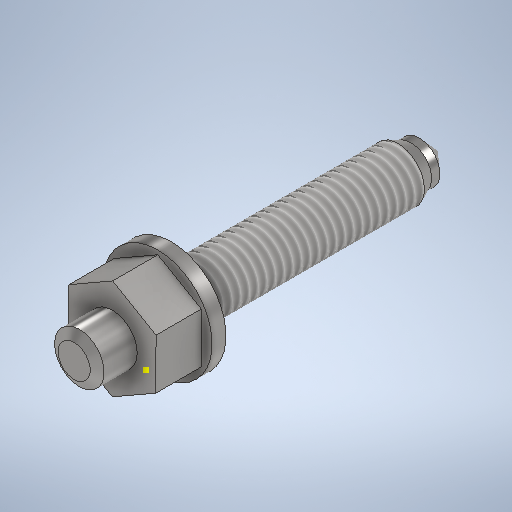
# Autodesk Inventor part: śróbki1
Saved by Autodesk Inventor 2025 (Build 290162000, 162)
## iProperties
Created: 2025-03-16
Part Number: śróbki1
Material: Stal nierdzewna
Document SubType Name: Modeling
Designer: barte
Density: 8 g/cm^3
Appearance: Częściowo polerowany
Author: barte
Autodesk Inventor part; units mm, degrees
ref_plane "YZ Plane" through (0, 0, 0) normal (1, 0, 0) x (0, 1, 0)
ref_plane "XZ Plane" through (0, 0, 0) normal (0, 1, 0) x (-1, 0, 0)
ref_plane "XY Plane" through (0, 0, 0) normal (0, 0, 1) x (1, 0, 0)
sketch "Szkic1" plane through (0, 0, 0) normal (0, 1, 0) x (-1, 0, 0)
  line L0 (0, 3.2611) -> (1.85, 3.2611)
  line L1 (1.85, 3.2611) -> (2.85, 2.6611)
  line L2 (2.85, 2.6611) -> (2.85, -6.3389)
  line L3 (2.85, -6.3389) -> (6.25, -6.3389)
  line L4 (6.25, -6.3389) -> (6.25, -7.9389)
  line L5 (6.25, -7.9389) -> (3.05, -7.9389)
  line L6 (3.05, -7.9389) -> (3.05, -33.9389)
  line L7 (3.05, -33.9389) -> (2.38, -35.4389)
  line L8 (2.38, -35.4389) -> (2.38, -36.3889)
  line L9 (2.38, -36.3889) -> (0, -38.5259)
  line L10 (0, 3.2611) -> (0, -38.5259)
  point P0 (0, 0)
  dimension "d0" = 1.85
  dimension "d1" = 0.6
  dimension "d2" = 1
  dimension "d3" = 9
  dimension "d4" = 3.4
  dimension "d5" = 1.6
  dimension "d6" = 3.2
  dimension "d7" = 26
  dimension "d8" = 1.5
  dimension "d9" = 0.67
  dimension "d10" = 0.95
  dimension "d11" = 2.137
  constraints: 22 end point, 3 perpendicular, 3 vertical, 2 horizontal
  measures "d0" distance of L0.start L0.end
  measures "d1" vertical distance of L0.end L1.end
  measures "d2" horizontal distance of L1.end L0.end
  measures "d3" distance of L1.end L2.end
  measures "d4" distance of L2.end L3.end
  measures "d5" distance of L3.end L4.end
  measures "d6" distance of L4.end L5.end
  measures "d7" distance of L5.end L6.end
  measures "d8" vertical distance of L6.end L7.end
  measures "d9" horizontal distance of L7.end L6.end
  measures "d10" distance of L7.end L8.end
  measures "d11" vertical distance of L9.end L8.end
revolve "Obrót1" add sketch "Szkic1" angle 360 about axis through (0, 0, 3.2611) along (0, 0, -1)
sketch "Szkic2" plane through (0, 0, -6.3389) normal (0, 0, 1) x (1, 0, 0)
  circle A0 centre (0, 0) radius 1.85 projected
  line L0 (5.0074, 2.8738) -> (4.9925, -2.8997)
  line L1 (4.9925, -2.8997) -> (-0.0149, -5.7735)
  line L2 (-0.0149, -5.7735) -> (-5.0074, -2.8738)
  line L3 (-5.0074, -2.8738) -> (-4.9925, 2.8997)
  line L4 (-4.9925, 2.8997) -> (0.0149, 5.7735)
  line L5 (0.0149, 5.7735) -> (5.0074, 2.8738)
  circle A1 centre (0, 0) radius 5
  point P0 (0, 0)
  dimension "d13" = 10
  constraints: 12 end point, 2 coincident, 1 centre point, 1 tangent, 13 other
  measures "d13" distance between parallel lines of L0 L3
sketch "Szkic3" plane through (0, 0, -7.9389) normal (0, 0, -1) x (-1, 0, 0)
  point P0 (0, 0)
extrude "Wyciągnięcie proste1" add sketch "Szkic2" along normal blind 5.2 contours A0 | L0 L1 A1 | L0 A1 L5 | A1 | A1 L4 L5 | L1 L2 A1 | A1 L3 L4 | L2 L3 A1
thread "Gwint1" size "M7x1" class "6g" standard "ANSI Metric M Profile" length 200
sketch "Szkic4" plane through (0, 0, -7.9389) normal (0, 0, -1) x (-1, 0, 0)
  point P0 (0, 0)
sketch "Szkic5" plane through (5.0074, 2.8738, -1.1389) normal (1, -0.0026, 0) x (0, 0, -1)
  point P0 (-1.1389, -2.8868)
sketch "Szkic6" plane through (0, 0, -7.9389) normal (0, 0, -1) x (-1, 0, 0)
  point P0 (0, 0)
sketch "Szkic7" plane through (5.0074, 2.8738, -1.1389) normal (1, -0.0026, 0) x (0, 0, -1)
  point P0 (-1.1389, -2.8868)
